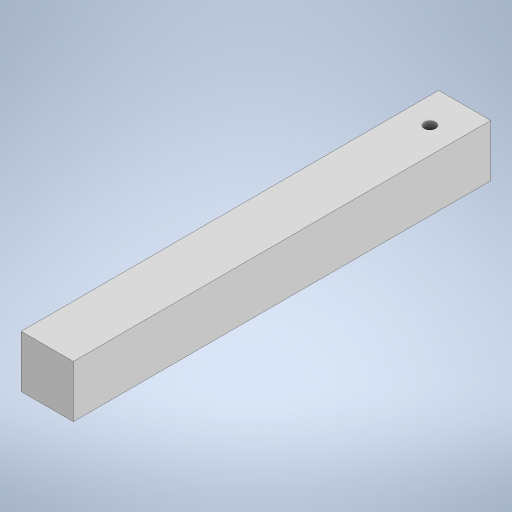
# Autodesk Inventor part: 射出_角柱7
Saved by Autodesk Inventor 2023 (Build 270158000, 158)
## iProperties
Created: 2022-04-20
Part Number: 射出_角柱7
Material: 一般
Document SubType Name: Modeling
Designer: yuta
Density: 1 g/cm^3
Appearance: 既定
Author: yuta
Autodesk Inventor part; units mm, degrees
ref_plane "YZ Plane" through (0, 0, 0) normal (1, 0, 0) x (0, 1, 0)
ref_plane "XZ Plane" through (0, 0, 0) normal (0, 1, 0) x (-1, 0, 0)
ref_plane "XY Plane" through (0, 0, 0) normal (0, 0, 1) x (1, 0, 0)
sketch "スケッチ1" plane through (0, 0, 0) normal (0, 0, 1) x (1, 0, 0)
  line L0 (0, 0) -> (15, 0)
  line L1 (15, 0) -> (15, 15)
  line L2 (15, 15) -> (0, 15)
  line L3 (0, 15) -> (0, 0)
  dimension "d0" = 15
  dimension "d1" = 15
  constraints: 8 end point, 2 parallel, 1 horizontal, 1 perpendicular
  measures "d0" distance of L2.end L1.end
  measures "d1" distance of L1.end L0.end
extrude "押し出し1" add sketch "スケッチ1" along normal blind 120
sketch "スケッチ2" plane through (0, 15, 0) normal (0, 1, 0) x (1, 0, 0)
  line L0 (15, 0) -> (0, 0) projected
  line L1 (15, 0) -> (15, -120) projected
  point P0 (7.5, -10)
  dimension "d4" = 10
  dimension "d5" = 7.5
  measures "d4" distance from line of L0 point (7.5, -10)
  measures "d5" distance from line of L1 point (7.5, -10)
hole "穴1" at (7.5, 15, 10) direction (0, -1, 0) diameter 3.2 end through all
